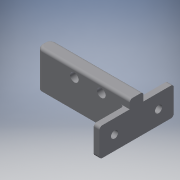
# Autodesk Inventor part: GuideArmConnector
Saved by Autodesk Inventor 2018 (Build 220112000, 112)
## iProperties
Created: 2017-12-14
Part Number: GuideArmConnector
Material: Generic
Document SubType Name: Modeling
Designer: reide
Density: 1 g/cm^3
Appearance: Default
Author: reide
Autodesk Inventor part; units mm, degrees
ref_plane "YZ Plane" through (0, 0, 0) normal (1, 0, 0) x (0, 1, 0)
ref_plane "XZ Plane" through (0, 0, 0) normal (0, 1, 0) x (-1, 0, 0)
sketch "Sketch1" plane through (0, 0, 0) normal (0, 0, 1) x (1, 0, 0)
  line L0 (-4.826, 0.413) -> (-4.826, -0.413) projected
  line L1 (-2.826, -2.413) -> (4.826, -2.413) projected
  line L2 (4.826, -2.413) -> (4.826, 2.413) projected
  line L3 (4.826, 2.413) -> (-2.826, 2.413) projected
  arc A0 (-4.826, -0.413) -> (-2.826, -2.413) centre (-2.826, -0.413) ccw projected
  arc A1 (-2.826, 2.413) -> (-4.826, 0.413) centre (-2.826, 0.413) ccw projected
  point P0 (0, 0)
extrude "Extrusion1" add sketch "Sketch1" along normal blind 10
sketch "Sketch2" plane through (4.826, -2.413, 0) normal (1, 0, 0) x (0, 0, -1)
  line L0 (0, 0) -> (-10, 0) projected
  line L1 (-10, 0) -> (-10, 4.826) projected
  circle A0 centre (3.175, 150.3292) radius 1.5 projected
  circle A1 centre (3.175, 23.749) radius 1.5 projected
  circle A2 centre (73.025, 23.749) radius 1.5 projected
  circle A3 centre (73.025, 150.3292) radius 1.5 projected
  arc A4 (60.2046, 236.2874) -> (0.9041, 211.5001) centre (77.9391, 110.5317) ccw projected
  ellipse E0 centre (170.686, 87.0391) end of major axis (408.43, 87.0391) minor radius 177.8 (0.9041, 211.5001) -> (0.9041, -37.4219) ccw projected
  arc A5 (0.9041, -37.4219) -> (60.2046, -62.2092) centre (77.9391, 63.5465) ccw projected
  arc A6 (60.2046, -62.2092) -> (281.1673, -62.2092) centre (170.686, 721.2179) ccw projected
  arc A7 (281.1673, -62.2092) -> (340.4678, -37.4219) centre (263.4329, 63.5465) ccw projected
  ellipse E1 centre (170.686, 87.0391) end of major axis (408.43, 87.0391) minor radius 177.8 (340.4678, -37.4219) -> (340.4678, 211.5001) ccw projected
  arc A8 (340.4678, 211.5001) -> (281.1673, 236.2874) centre (263.4329, 110.5317) ccw projected
  arc A9 (281.1673, 236.2874) -> (60.2046, 236.2874) centre (170.686, -547.1397) ccw projected
  circle A10 centre (18.1159, 118.5546) radius 1.25 projected
  circle A11 centre (-51.7341, 53.7756) radius 1.25 projected
  circle A12 centre (18.1159, 53.7756) radius 1.25 projected
  circle A13 centre (-51.7341, 118.5546) radius 1.25 projected
  circle A14 centre (395.605, 77.7641) radius 1.25 projected
  circle A15 centre (321.1037, 62.7821) radius 1.25 projected
  circle A16 centre (321.1037, 101.1361) radius 1.25 projected
  circle A17 centre (395.605, 96.3141) radius 1.25 projected
  line L2 (284.5488, 72.0792) -> (223.628, 72.0792) projected
  line L3 (223.628, 72.0792) -> (223.628, 102.5592) projected
  line L4 (223.628, 102.5592) -> (284.5488, 102.5592) projected
  line L5 (284.5488, 102.5592) -> (284.5488, 72.0792) projected
  circle A18 centre (129.4087, 87.0391) radius 30.4 projected
  line L6 (95.6616, 45.3432) -> (95.6616, 49.3432) projected
  arc A19 (98.6614, 49.3432) -> (95.6616, 49.3432) centre (97.1615, 49.3432) ccw projected
  line L7 (98.6614, 49.3432) -> (98.6614, 45.3432) projected
  arc A20 (95.6616, 45.3432) -> (98.6614, 45.3432) centre (97.1615, 45.3432) ccw projected
  line L8 (160.3503, 45.3892) -> (160.3503, 49.3892) projected
  arc A21 (163.3501, 49.3892) -> (160.3503, 49.3892) centre (161.8502, 49.3892) ccw projected
  line L9 (163.3501, 49.3892) -> (163.3501, 45.3892) projected
  arc A22 (160.3503, 45.3892) -> (163.3501, 45.3892) centre (161.8502, 45.3892) ccw projected
  line L10 (95.5803, 159.8921) -> (95.5803, 163.8921) projected
  arc A23 (98.5801, 163.8921) -> (95.5803, 163.8921) centre (97.0802, 163.8921) ccw projected
  line L11 (98.5801, 163.8921) -> (98.5801, 159.8921) projected
  arc A24 (95.5803, 159.8921) -> (98.5801, 159.8921) centre (97.0802, 159.8921) ccw projected
  line L12 (163.3504, 163.8921) -> (163.3504, 159.8921) projected
  arc A25 (160.3506, 159.8921) -> (163.3504, 159.8921) centre (161.8505, 159.8921) ccw projected
  line L13 (160.3506, 159.8921) -> (160.3506, 163.8921) projected
  arc A26 (163.3504, 163.8921) -> (160.3506, 163.8921) centre (161.8505, 163.8921) ccw projected
  arc A27 (180.3755, 134.9774) -> (180.3753, 131.9798) centre (180.3755, 133.4786) ccw projected
  line L14 (180.3755, 134.9774) -> (184.3754, 134.9776) projected
  arc A28 (184.3754, 131.9796) -> (184.3754, 134.9776) centre (184.3755, 133.4786) ccw projected
  line L15 (184.3754, 131.9796) -> (180.3753, 131.9798) projected
  arc A29 (65.9852, 134.9725) -> (65.9851, 131.9749) centre (65.9852, 133.4737) ccw projected
  line L16 (65.9852, 134.9725) -> (69.9852, 134.9727) projected
  arc A30 (69.9852, 131.9747) -> (69.9852, 134.9727) centre (69.9852, 133.4737) ccw projected
  line L17 (69.9852, 131.9747) -> (65.9851, 131.9749) projected
  arc A31 (188.0254, 134.9778) -> (188.0255, 131.9802) centre (188.0255, 133.479) ccw projected
  line L18 (188.0254, 134.9778) -> (192.0254, 134.978) projected
  arc A32 (192.0254, 131.98) -> (192.0254, 134.978) centre (192.0255, 133.479) ccw projected
  line L19 (192.0254, 131.98) -> (188.0255, 131.9802) projected
  arc A33 (73.6382, 70.1265) -> (73.6381, 67.1289) centre (73.6382, 68.6277) ccw projected
  line L20 (73.6382, 70.1265) -> (77.6381, 70.1267) projected
  arc A34 (77.6381, 67.1287) -> (77.6381, 70.1267) centre (77.6382, 68.6277) ccw projected
  line L21 (77.6381, 67.1287) -> (73.6381, 67.1289) projected
  circle A35 centre (271.4412, 59.8872) radius 1.25 projected
  circle A36 centre (229.978, 118.4342) radius 1.25 projected
  circle A37 centre (281.3738, 108.9092) radius 1.25 projected
  circle A38 centre (278.1988, 118.4342) radius 1.25 projected
  circle A39 centre (254.0826, 118.4342) radius 1.25 projected
  circle A40 centre (226.803, 108.9092) radius 1.25 projected
  circle A41 centre (226.5872, 59.8872) radius 1.25 projected
  arc A42 (188.0714, 70.2078) -> (188.0714, 67.2102) centre (188.0714, 68.709) ccw projected
  line L22 (188.0714, 70.2078) -> (192.0714, 70.208) projected
  arc A43 (192.0714, 67.21) -> (192.0714, 70.208) centre (192.0714, 68.709) ccw projected
  line L23 (192.0714, 67.21) -> (188.0714, 67.2102) projected
  line L24 (73.6352, 134.9725) -> (77.6351, 134.9727) projected
  arc A44 (77.6351, 131.9747) -> (77.6351, 134.9727) centre (77.6352, 133.4737) ccw projected
  line L25 (77.6351, 131.9747) -> (73.6351, 131.9749) projected
  arc A45 (73.6352, 134.9725) -> (73.6351, 131.9749) centre (73.6352, 133.4737) ccw projected
  arc A46 (66.0312, 70.1211) -> (66.0311, 67.1235) centre (66.0312, 68.6223) ccw projected
  line L26 (66.0312, 70.1211) -> (70.0312, 70.1213) projected
  arc A47 (70.0312, 67.1233) -> (70.0312, 70.1213) centre (70.0312, 68.6223) ccw projected
  line L27 (70.0312, 67.1233) -> (66.0311, 67.1235) projected
  arc A48 (180.4215, 70.2024) -> (180.4213, 67.2048) centre (180.4215, 68.7036) ccw projected
  line L28 (180.4215, 70.2024) -> (184.4214, 70.2025) projected
  arc A49 (184.4214, 67.2046) -> (184.4214, 70.2025) centre (184.4215, 68.7036) ccw projected
  line L29 (184.4214, 67.2046) -> (180.4213, 67.2048) projected
  line L30 (160.3503, 152.2421) -> (160.3503, 156.2421) projected
  arc A50 (163.3501, 156.2421) -> (160.3503, 156.2421) centre (161.8502, 156.2421) ccw projected
  line L31 (163.3501, 156.2421) -> (163.3501, 152.2421) projected
  arc A51 (160.3503, 152.2421) -> (163.3501, 152.2421) centre (161.8502, 152.2421) ccw projected
  line L32 (95.5857, 152.1961) -> (95.5857, 156.1961) projected
  arc A52 (98.5855, 156.1961) -> (95.5857, 156.1961) centre (97.0856, 156.1961) ccw projected
  line L33 (98.5855, 156.1961) -> (98.5855, 152.1961) projected
  arc A53 (95.5857, 152.1961) -> (98.5855, 152.1961) centre (97.0856, 152.1961) ccw projected
  line L34 (160.3503, 37.7392) -> (160.3503, 41.7392) projected
  arc A54 (163.3501, 41.7392) -> (160.3503, 41.7392) centre (161.8502, 41.7392) ccw projected
  line L35 (163.3501, 41.7392) -> (163.3501, 37.7392) projected
  arc A55 (160.3503, 37.7392) -> (163.3501, 37.7392) centre (161.8502, 37.7392) ccw projected
  line L36 (95.667, 37.6932) -> (95.667, 41.6932) projected
  arc A56 (98.6669, 41.6932) -> (95.667, 41.6932) centre (97.167, 41.6932) ccw projected
  line L37 (98.6669, 41.6932) -> (98.6669, 37.6932) projected
  arc A57 (95.667, 37.6932) -> (98.6669, 37.6932) centre (97.167, 37.6932) ccw projected
  line L38 (0, 4.826) -> (-10, 4.826) projected
  line L39 (0, -10.668) -> (0, 15.494) projected
  circle A58 centre (-5, -5.334) radius 1.5 projected
  circle A59 centre (81.2, -5.334) radius 1.5 projected
  circle A60 centre (81.2, 10.16) radius 1.5 projected
  circle A61 centre (-5, 10.16) radius 1.5 projected
  circle A62 centre (-5, 163.9182) radius 1.5 projected
  circle A63 centre (81.2, 163.9182) radius 1.5 projected
  circle A64 centre (81.2, 179.4122) radius 1.5 projected
  circle A65 centre (-5, 179.4122) radius 1.5 projected
  circle A66 centre (73.025, 187.9212) radius 1.5 projected
  circle A67 centre (73.025, -13.843) radius 1.5 projected
  circle A68 centre (3.175, -13.843) radius 1.5 projected
  circle A69 centre (3.175, 187.9212) radius 1.5 projected
  circle A70 centre (268.3469, 187.9212) radius 1.5 projected
  circle A71 centre (260.1719, 179.4122) radius 1.5 projected
  circle A72 centre (346.3719, 10.16) radius 1.5 projected
  circle A73 centre (346.3719, -5.334) radius 1.5 projected
  circle A74 centre (346.3719, 179.4122) radius 1.5 projected
  circle A75 centre (338.1969, 150.3292) radius 1.5 projected
  circle A76 centre (260.1719, -5.334) radius 1.5 projected
  circle A77 centre (268.3469, 23.749) radius 1.5 projected
  circle A78 centre (268.3469, -13.843) radius 1.5 projected
  circle A79 centre (260.1719, 10.16) radius 1.5 projected
  circle A80 centre (268.3469, 150.3292) radius 1.5 projected
  circle A81 centre (338.1969, -13.843) radius 1.5 projected
  circle A82 centre (338.1969, 23.749) radius 1.5 projected
  circle A83 centre (260.1719, 163.9182) radius 1.5 projected
  circle A84 centre (338.1969, 187.9212) radius 1.5 projected
  circle A85 centre (346.3719, 163.9182) radius 1.25 projected
  point P0 (0, 2.413)
  constraints: 2 other
ref_plane "Work Plane1" through (27.9676, -72.374, -408.43) normal (-1, 0, 0) x (0, 0, 1)
extrude "Extrusion2" add sketch "Sketch2" along normal up to surface (23.1416 mm away) contours L0 L1 L38 L39
sketch "Sketch3" plane through (27.9676, -2.413, 10) normal (1, 0, 0) x (0, 0, -1)
  line L0 (10, -10.668) -> (10, 15.494) projected
  line L1 (10, -10.668) -> (0, -10.668)
  line L2 (0, -10.668) -> (0, 15.494)
  line L3 (0, 15.494) -> (10, 15.494)
  line L4 (10, 15.494) -> (10, -10.668)
  line L5 (10, 2.826) -> (10, 2) projected
  line L6 (10, 0) -> (10, -10.668)
  line L7 (10, 4.826) -> (10, 15.494)
  circle A0 centre (5, -5.334) radius 1.25
  circle A1 centre (5, 10.16) radius 1.25
  point P0 (10, 2.413)
  point P1 (5, -10.668)
  point P2 (5, 15.494)
  point P3 (10, -5.334)
  point P4 (10, 10.16)
  dimension "d4" = 2.5
  dimension "d5" = 2.5
  constraints: 12 end point, 4 midpoint, 2 centre point, 2 parallel, 2 perpendicular, 1 collinear, 1 horizontal
  measures "d4" diameter of A0
  measures "d5" diameter of A1
extrude "Extrusion3" add sketch "Sketch3" against normal blind 2
fillet "Fillet1" radius 1 6 edges at (25.9676, -2.413, 5) (25.9676, 2.413, 5) (26.9676, 13.081, 0) (26.9676, 13.081, 10) (26.9676, -13.081, 10) (26.9676, -13.081, 0)
sketch "Sketch4" plane through (0, 0, 10) normal (0, 0, 1) x (1, 0, 0)
  point P0 (0, 0)
sketch "Sketch5" plane through (0, 0, 10) normal (0, 0, 1) x (1, 0, 0)
  line L0 (27.9676, -12.081) -> (25.9676, -12.081) projected
  line L1 (27.9676, 12.081) -> (27.9676, -12.081) projected
  line L2 (25.9676, 12.081) -> (27.9676, 12.081) projected
  line L3 (25.9676, 3.413) -> (25.9676, 12.081) projected
  arc A0 (24.9676, 2.413) -> (25.9676, 3.413) centre (24.9676, 3.413) ccw projected
  line L4 (-2.826, 2.413) -> (24.9676, 2.413) projected
  arc A1 (-2.826, 2.413) -> (-4.826, 0.413) centre (-2.826, 0.413) ccw projected
  line L5 (-4.826, 0.413) -> (-4.826, -0.413) projected
  arc A2 (-4.826, -0.413) -> (-2.826, -2.413) centre (-2.826, -0.413) ccw projected
  line L6 (-2.826, -2.413) -> (24.9676, -2.413) projected
  arc A3 (25.9676, -3.413) -> (24.9676, -2.413) centre (24.9676, -3.413) ccw projected
  line L7 (25.9676, -12.081) -> (25.9676, -3.413) projected
  line L8 (-2.826, 2.413) -> (24.9676, 2.413) projected
  line L9 (-2.826, 2.413) -> (27.9676, 2.413)
  line L10 (27.9676, 2.413) -> (27.9676, -2.413)
  line L11 (27.9676, -2.413) -> (-2.826, -2.413)
  line L12 (-2.826, -2.413) -> (-2.826, 2.413)
  circle A4 centre (-2.826, 0.413) radius 2
  circle A5 centre (-2.826, -0.413) radius 2
  line L13 (-4.826, 0.413) -> (-4.826, -0.413) projected
  line L14 (-4.826, -0.413) -> (-4.826, 0.413)
  arc A6 (-2.826, 2.413) -> (-4.826, 0.413) centre (-2.826, 0.413) ccw projected
  point P0 (0, 0)
  constraints: 10 end point, 2 coincident, 2 parallel, 1 centre point, 1 horizontal, 1 perpendicular, 1 point on circle, 1 point on line, 1 tangent, 1 vertical, 1 vertical alignment, 2 other
extrude "Extrusion4" add sketch "Sketch5" along normal blind 3 contours L11 L6 A5 A4 L4 L9 L1 | A2 A5 A4 L12 | L12 A4 A5 | L12 A5 A4 A1 | A4 A5 L12 | A4 A5 L12 | L12 A5 A4
sketch "Sketch6" plane through (-2.826, -2.413, 0) normal (0, -1, 0) x (1, 0, 0)
  line L0 (30.7936, 13) -> (0, 13) projected
  line L1 (30.7936, 10) -> (30.7936, 13) projected
  line L2 (30.7936, 13) -> (30.7936, 10)
  line L3 (30.7936, 10) -> (20.7936, 10)
  circle A0 centre (20.7936, 10) radius 1.5
  line L4 (20.7936, 10) -> (11.2936, 10)
  circle A1 centre (11.2936, 10) radius 1.5
  point P0 (2.826, 0)
  dimension "d11" = 10
  dimension "d12" = 3
  dimension "d13" = 9.5
  dimension "d14" = 3
  constraints: 6 end point, 2 centre point, 2 coincident, 1 horizontal, 1 perpendicular, 1 vertical
  measures "d11" distance of L1.start L3.end
  measures "d12" diameter of A0
  measures "d13" distance of L4.start L4.end
  measures "d14" diameter of A1
extrude "Extrusion5" cut sketch "Sketch6" against normal blind 100
fillet "Fillet2" radius 1 4 edges at (12.5708, -2.413, 13) (-4.3794, -1.6728, 13) (12.5708, 2.413, 13) (-4.3794, 1.6728, 13)
body "Solid1"
